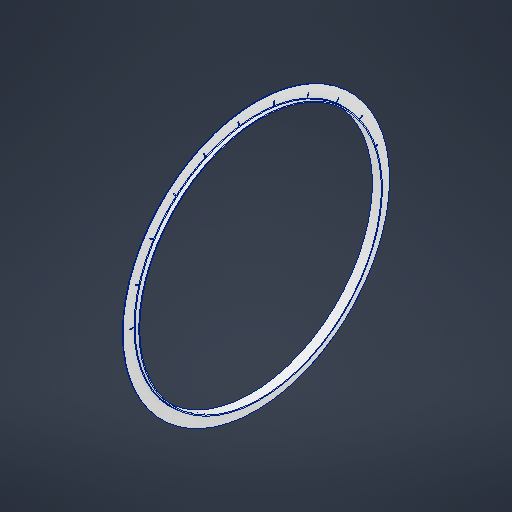
# Autodesk Inventor part: Support Ring, T-Section
Saved by Autodesk Inventor 2026 (Build 300175000, 175)
## iProperties
Created: 2025-11-01
Part Number: Support Ring, T-Section
Material: Aluminum 6061
Document SubType Name: Modeling
Designer: Brandon Portillo
Density: 2.7 g/cm^3
Appearance: Aluminum - Flat
Author: Brandon Portillo
Autodesk Inventor part; units mm, degrees
ref_plane "YZ Plane" through (0, 0, 0) normal (1, 0, 0) x (0, 1, 0)
ref_plane "XZ Plane" through (0, 0, 0) normal (0, 1, 0) x (-1, 0, 0)
ref_plane "XY Plane" through (0, 0, 0) normal (0, 0, 1) x (1, 0, 0)
sketch "Sketch1" plane through (0, 0, 0) normal (0, 1, 0) x (-1, 0, 0)
  line L0 (0, 0) -> (-10, 0)
  line L1 (-10, 0) -> (-10, -172)
  line L2 (0, -172) -> (0, 0)
  line L3 (8, -180) -> (65, -180)
  line L4 (65, -180) -> (65, -195)
  line L5 (65, -195) -> (-5, -195)
  line L6 (-18, -180) -> (-75, -180)
  line L7 (-75, -180) -> (-75, -195)
  line L8 (-75, -195) -> (-5, -195)
  arc A0 (0, -172) -> (8, -180) centre (8, -172) ccw
  arc A1 (-18, -180) -> (-10, -172) centre (-18, -172) ccw
  line L9 (-5, -195) -> (0, -2089.9934)
  line L10 (0, -2089.9934) -> (299.999, -2089.2018)
  point P0 (0, -180)
  point P1 (-10, -180)
  dimension "d4" = 15
  dimension "d5" = 180
  dimension "d6" = 10
  dimension "d7" = 65
  dimension "d8" = 8
  dimension "d9" = 8
  dimension "d10" = 1895
  dimension "d11" = 300
  constraints: 22 end point, 5 point on line, 4 point on circle, 4 tangent, 3 perpendicular, 2 centre point, 2 horizontal, 2 parallel
  measures "d4" distance of L3.end L4.end
  measures "d5" distance of L0.end point (-10, -180)
  measures "d6" distance of L0.start L0.end
  measures "d7" distance of point (0, -180) L3.end
  measures "d8" radius of A0
  measures "d9" radius of A1
  measures "d10" distance of L5.end L9.end
  measures "d11" distance of L9.end L10.end
revolve "Revolution1" add sketch "Sketch1" angle 360 about axis through (0, 0, -2089.9934) along (-0.9999965, 0, 0.0026385)
sketch "Sketch2" plane through (0, 0, 0) normal (1, 0, 0) x (0, 1, 0)
  line L0 (0, 0) -> (0, -135)
  line L1 (0, -155) -> (0, -115) construction
  line L2 (6.5, -155) -> (6.5, -115)
  line L3 (-6.5, -115) -> (-6.5, -155)
  arc A0 (-6.5, -155) -> (6.5, -155) centre (0, -155) ccw
  arc A1 (6.5, -115) -> (-6.5, -115) centre (0, -115) ccw
  ellipse E0 centre (0, -2090.0064) end of major axis (1918.0131, -2090.0064) minor radius 1918.0064 projected
  ellipse E1 centre (0, -2090.0052) end of major axis (2090.0125, -2090.0052) minor radius 2090.0052 projected
  ellipse E2 centre (0, -2090.0064) end of major axis (1918.0131, -2090.0064) minor radius 1918.0064 projected
  circle A2 centre (0, -2090.0064) radius 1895.0064
  ellipse E3 centre (0, -2090.1781) end of major axis (1895.1847, -2090.1781) minor radius 1895.1781 projected
  line L4 (-500.8165, -220.9337) -> (-511.1693, -182.2967) construction
  line L5 (-494.538, -219.2514) -> (-504.8908, -180.6144)
  line L6 (-517.4478, -183.979) -> (-507.095, -222.6161)
  arc A3 (-507.095, -222.6161) -> (-494.538, -219.2514) centre (-500.8165, -220.9337) ccw
  arc A4 (-504.8908, -180.6144) -> (-517.4478, -183.979) centre (-511.1693, -182.2967) ccw
  line L7 (-967.5032, -414.2417) -> (-987.5032, -379.6007) construction
  line L8 (-961.8741, -410.9917) -> (-981.8741, -376.3507)
  line L9 (-993.1324, -382.8507) -> (-973.1324, -417.4917)
  arc A5 (-973.1324, -417.4917) -> (-961.8741, -410.9917) centre (-967.5032, -414.2417) ccw
  arc A6 (-981.8741, -376.3507) -> (-993.1324, -382.8507) centre (-987.5032, -379.6007) ccw
  line L10 (-1368.2562, -721.7503) -> (-1396.5404, -693.466) construction
  line L11 (-1363.66, -717.1541) -> (-1391.9442, -688.8698)
  line L12 (-1401.1366, -698.0622) -> (-1372.8524, -726.3465)
  arc A7 (-1372.8524, -726.3465) -> (-1363.66, -717.1541) centre (-1368.2562, -721.7503) ccw
  arc A8 (-1391.9442, -688.8698) -> (-1401.1366, -698.0622) centre (-1396.5404, -693.466) ccw
  line L13 (-1675.7647, -1122.5032) -> (-1710.4057, -1102.5032) construction
  line L14 (-1672.5147, -1116.8741) -> (-1707.1557, -1096.8741)
  line L15 (-1713.6557, -1108.1324) -> (-1679.0147, -1128.1324)
  arc A9 (-1679.0147, -1128.1324) -> (-1672.5147, -1116.8741) centre (-1675.7647, -1122.5032) ccw
  arc A10 (-1707.1557, -1096.8741) -> (-1713.6557, -1108.1324) centre (-1710.4057, -1102.5032) ccw
  line L16 (-1869.0727, -1589.1899) -> (-1907.7097, -1578.8372) construction
  line L17 (-1867.3904, -1582.9114) -> (-1906.0274, -1572.5586)
  line L18 (-1909.392, -1585.1157) -> (-1870.755, -1595.4684)
  arc A11 (-1870.755, -1595.4684) -> (-1867.3904, -1582.9114) centre (-1869.0727, -1589.1899) ccw
  arc A12 (-1906.0274, -1572.5586) -> (-1909.392, -1585.1157) centre (-1907.7097, -1578.8372) ccw
  line L19 (-1935.0064, -2090.0064) -> (-1975.0064, -2090.0064) construction
  line L20 (-1935.0064, -2083.5064) -> (-1975.0064, -2083.5064)
  line L21 (-1975.0064, -2096.5064) -> (-1935.0064, -2096.5064)
  arc A13 (-1935.0064, -2096.5064) -> (-1935.0064, -2083.5064) centre (-1935.0064, -2090.0064) ccw
  arc A14 (-1975.0064, -2083.5064) -> (-1975.0064, -2096.5064) centre (-1975.0064, -2090.0064) ccw
  line L22 (-1869.0727, -2590.823) -> (-1907.7097, -2601.1757) construction
  line L23 (-1870.755, -2584.5444) -> (-1909.392, -2594.8972)
  line L24 (-1906.0274, -2607.4542) -> (-1867.3904, -2597.1015)
  arc A15 (-1867.3904, -2597.1015) -> (-1870.755, -2584.5444) centre (-1869.0727, -2590.823) ccw
  arc A16 (-1909.392, -2594.8972) -> (-1906.0274, -2607.4542) centre (-1907.7097, -2601.1757) ccw
  line L25 (-1675.7647, -3057.5097) -> (-1710.4057, -3077.5097) construction
  line L26 (-1679.0147, -3051.8805) -> (-1713.6557, -3071.8805)
  line L27 (-1707.1557, -3083.1388) -> (-1672.5147, -3063.1388)
  arc A17 (-1672.5147, -3063.1388) -> (-1679.0147, -3051.8805) centre (-1675.7647, -3057.5097) ccw
  arc A18 (-1713.6557, -3071.8805) -> (-1707.1557, -3083.1388) centre (-1710.4057, -3077.5097) ccw
  line L28 (-1368.2562, -3458.2626) -> (-1396.5404, -3486.5469) construction
  line L29 (-1372.8524, -3453.6664) -> (-1401.1366, -3481.9507)
  line L30 (-1391.9442, -3491.1431) -> (-1363.66, -3462.8588)
  arc A19 (-1363.66, -3462.8588) -> (-1372.8524, -3453.6664) centre (-1368.2562, -3458.2626) ccw
  arc A20 (-1401.1366, -3481.9507) -> (-1391.9442, -3491.1431) centre (-1396.5404, -3486.5469) ccw
  line L31 (-967.5032, -3765.7712) -> (-987.5032, -3800.4122) construction
  line L32 (-973.1324, -3762.5212) -> (-993.1324, -3797.1622)
  line L33 (-981.8741, -3803.6622) -> (-961.8741, -3769.0212)
  arc A21 (-961.8741, -3769.0212) -> (-973.1324, -3762.5212) centre (-967.5032, -3765.7712) ccw
  arc A22 (-993.1324, -3797.1622) -> (-981.8741, -3803.6622) centre (-987.5032, -3800.4122) ccw
  line L34 (-500.8165, -3959.0791) -> (-511.1693, -3997.7162) construction
  line L35 (-507.095, -3957.3968) -> (-517.4478, -3996.0338)
  line L36 (-504.8908, -3999.3985) -> (-494.538, -3960.7615)
  arc A23 (-494.538, -3960.7615) -> (-507.095, -3957.3968) centre (-500.8165, -3959.0791) ccw
  arc A24 (-517.4478, -3996.0338) -> (-504.8908, -3999.3985) centre (-511.1693, -3997.7162) ccw
  line L37 (0, -4025.0129) -> (0, -4065.0129) construction
  line L38 (-6.5, -4025.0129) -> (-6.5, -4065.0129)
  line L39 (6.5, -4065.0129) -> (6.5, -4025.0129)
  arc A25 (6.5, -4025.0129) -> (-6.5, -4025.0129) centre (0, -4025.0129) ccw
  arc A26 (-6.5, -4065.0129) -> (6.5, -4065.0129) centre (0, -4065.0129) ccw
  line L40 (500.8165, -3959.0791) -> (511.1693, -3997.7162) construction
  line L41 (494.538, -3960.7615) -> (504.8908, -3999.3985)
  line L42 (517.4478, -3996.0338) -> (507.095, -3957.3968)
  arc A27 (507.095, -3957.3968) -> (494.538, -3960.7615) centre (500.8165, -3959.0791) ccw
  arc A28 (504.8908, -3999.3985) -> (517.4478, -3996.0338) centre (511.1693, -3997.7162) ccw
  line L43 (967.5032, -3765.7712) -> (987.5032, -3800.4122) construction
  line L44 (961.8741, -3769.0212) -> (981.8741, -3803.6622)
  line L45 (993.1324, -3797.1622) -> (973.1324, -3762.5212)
  arc A29 (973.1324, -3762.5212) -> (961.8741, -3769.0212) centre (967.5032, -3765.7712) ccw
  arc A30 (981.8741, -3803.6622) -> (993.1324, -3797.1622) centre (987.5032, -3800.4122) ccw
  line L46 (1368.2562, -3458.2626) -> (1396.5404, -3486.5469) construction
  line L47 (1363.66, -3462.8588) -> (1391.9442, -3491.1431)
  line L48 (1401.1366, -3481.9507) -> (1372.8524, -3453.6664)
  arc A31 (1372.8524, -3453.6664) -> (1363.66, -3462.8588) centre (1368.2562, -3458.2626) ccw
  arc A32 (1391.9442, -3491.1431) -> (1401.1366, -3481.9507) centre (1396.5404, -3486.5469) ccw
  line L49 (1675.7647, -3057.5097) -> (1710.4057, -3077.5097) construction
  line L50 (1672.5147, -3063.1388) -> (1707.1557, -3083.1388)
  line L51 (1713.6557, -3071.8805) -> (1679.0147, -3051.8805)
  arc A33 (1679.0147, -3051.8805) -> (1672.5147, -3063.1388) centre (1675.7647, -3057.5097) ccw
  arc A34 (1707.1557, -3083.1388) -> (1713.6557, -3071.8805) centre (1710.4057, -3077.5097) ccw
  line L52 (1869.0727, -2590.823) -> (1907.7097, -2601.1757) construction
  line L53 (1867.3904, -2597.1015) -> (1906.0274, -2607.4542)
  line L54 (1909.392, -2594.8972) -> (1870.755, -2584.5444)
  arc A35 (1870.755, -2584.5444) -> (1867.3904, -2597.1015) centre (1869.0727, -2590.823) ccw
  arc A36 (1906.0274, -2607.4542) -> (1909.392, -2594.8972) centre (1907.7097, -2601.1757) ccw
  line L55 (1935.0064, -2090.0064) -> (1975.0064, -2090.0064) construction
  line L56 (1935.0064, -2096.5064) -> (1975.0064, -2096.5064)
  line L57 (1975.0064, -2083.5064) -> (1935.0064, -2083.5064)
  arc A37 (1935.0064, -2083.5064) -> (1935.0064, -2096.5064) centre (1935.0064, -2090.0064) ccw
  arc A38 (1975.0064, -2096.5064) -> (1975.0064, -2083.5064) centre (1975.0064, -2090.0064) ccw
  line L58 (1869.0727, -1589.1899) -> (1907.7097, -1578.8372) construction
  line L59 (1870.755, -1595.4684) -> (1909.392, -1585.1157)
  line L60 (1906.0274, -1572.5586) -> (1867.3904, -1582.9114)
  arc A39 (1867.3904, -1582.9114) -> (1870.755, -1595.4684) centre (1869.0727, -1589.1899) ccw
  arc A40 (1909.392, -1585.1157) -> (1906.0274, -1572.5586) centre (1907.7097, -1578.8372) ccw
  line L61 (1675.7647, -1122.5032) -> (1710.4057, -1102.5032) construction
  line L62 (1679.0147, -1128.1324) -> (1713.6557, -1108.1324)
  line L63 (1707.1557, -1096.8741) -> (1672.5147, -1116.8741)
  arc A41 (1672.5147, -1116.8741) -> (1679.0147, -1128.1324) centre (1675.7647, -1122.5032) ccw
  arc A42 (1713.6557, -1108.1324) -> (1707.1557, -1096.8741) centre (1710.4057, -1102.5032) ccw
  line L64 (1368.2562, -721.7503) -> (1396.5404, -693.466) construction
  line L65 (1372.8524, -726.3465) -> (1401.1366, -698.0622)
  line L66 (1391.9442, -688.8698) -> (1363.66, -717.1541)
  arc A43 (1363.66, -717.1541) -> (1372.8524, -726.3465) centre (1368.2562, -721.7503) ccw
  arc A44 (1401.1366, -698.0622) -> (1391.9442, -688.8698) centre (1396.5404, -693.466) ccw
  line L67 (967.5032, -414.2417) -> (987.5032, -379.6007) construction
  line L68 (973.1324, -417.4917) -> (993.1324, -382.8507)
  line L69 (981.8741, -376.3507) -> (961.8741, -410.9917)
  arc A45 (961.8741, -410.9917) -> (973.1324, -417.4917) centre (967.5032, -414.2417) ccw
  arc A46 (993.1324, -382.8507) -> (981.8741, -376.3507) centre (987.5032, -379.6007) ccw
  line L70 (500.8165, -220.9337) -> (511.1693, -182.2967) construction
  line L71 (507.095, -222.6161) -> (517.4478, -183.979)
  line L72 (504.8908, -180.6144) -> (494.538, -219.2514)
  arc A47 (494.538, -219.2514) -> (507.095, -222.6161) centre (500.8165, -220.9337) ccw
  arc A48 (517.4478, -183.979) -> (504.8908, -180.6144) centre (511.1693, -182.2967) ccw
  point P0 (-505.9929, -201.6152)
  point P1 (-977.5032, -396.9212)
  point P2 (-1382.3983, -707.6081)
  point P3 (-1693.0852, -1112.5032)
  point P4 (-1888.3912, -1584.0135)
  point P5 (-1955.0064, -2090.0064)
  point P6 (-1888.3912, -2595.9993)
  point P7 (-1693.0852, -3067.5097)
  point P8 (-1382.3983, -3472.4047)
  point P9 (-977.5032, -3783.0917)
  point P10 (-505.9929, -3978.3976)
  point P11 (0, -4045.0129)
  point P12 (505.9929, -3978.3976)
  point P13 (977.5032, -3783.0917)
  point P14 (1382.3983, -3472.4047)
  point P15 (1693.0852, -3067.5097)
  point P16 (1888.3912, -2595.9993)
  point P17 (1955.0064, -2090.0064)
  point P18 (1888.3912, -1584.0135)
  point P19 (1693.0852, -1112.5032)
  point P20 (1382.3983, -707.6081)
  point P21 (977.5032, -396.9212)
  point P22 (505.9929, -201.6152)
  dimension "d13" = 135
  dimension "d14" = 20
  dimension "d15" = 13
  dimension "d18" = 360
  constraints: 194 end point, 96 point on circle, 49 centre point, 4 tangent, 1 coincident, 1 midpoint, 1 parallel, 1 point on line, 1 vertical, 290 other
  measures "d13" distance of L0.start L0.end
  measures "d14" distance of L0.end L1.end
  measures "d15" diameter of A1
extrude "Extrusion1" cut sketch "Sketch2" along normal mid plane 20 contours A0 L3 A1 L2
pattern_circular "Circular Pattern1" count 12 over 180 about axis through (69.9797, 0, -2090.178) along (-0.9999965, 0, 0.0026385) of "Extrusion1"
body "Solid1"
